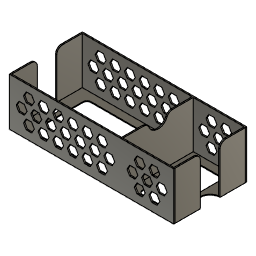
Food_Chain_Magnate_Card_Holder v2 (Autodesk Fusion 360 design; units mm, degrees)
Autodesk Fusion 360 part; units mm, degrees
sketch "Sketch1" plane through (0, 0, 0) normal (0, 0, 1) x (1, 0, 0)
  line L0 (-50, 26.6) -> (160, 26.6)
  line L1 (-50, 26.6) -> (-50, 25)
  line L2 (160, 26.6) -> (160, 25)
  line L3 (159.9999, -66.6) -> (-50, -66.6)
  line L4 (-50, -66.6) -> (-50, -65)
  line L5 (159.9999, -66.6) -> (160, -65)
  line L6 (-48.4, -64.9241) -> (-48.4, -65)
  line L7 (93.4, 25) -> (93.4, -65)
  line L8 (91.8, 25) -> (91.8, -65)
  line L9 (-48.4, 25) -> (91.8, 25)
  line L10 (93.4, 25) -> (158.4, 25)
  line L11 (158.4, -65) -> (93.4, -65)
  line L12 (91.8, -65) -> (-48.4, -65)
  line L13 (103.4, 10) -> (103.4, -50)
  line L14 (137.4, -55) -> (108.4, -55)
  line L15 (108.4, 15) -> (137.4, 15)
  line L16 (76.8, -55) -> (-27.4, -55)
  line L17 (81.8, 10) -> (81.8, -50)
  line L18 (-27.4, 15) -> (76.8, 15)
  line L19 (-32.4, 10) -> (-32.4, -50)
  line L20 (142.4, 10) -> (142.4, -50)
  arc A0 (-50, -32.5) -> (-50, -7.5) centre (-50, -20) ccw
  line L21 (-50, -65) -> (-50, -32.5)
  line L22 (-50, -7.5) -> (-50, 25)
  line L23 (-48.4, 25) -> (-48.4, -7.6028)
  line L24 (-48.4, -32.3972) -> (-48.4, -65)
  arc A1 (160, -7.5) -> (160, -32.5) centre (160, -20) ccw
  line L25 (160, 25) -> (160, -7.5)
  line L26 (160, -32.5) -> (160, -65)
  line L27 (158.4, 25) -> (158.4, -7.6028)
  line L28 (158.4, -32.3972) -> (158.4, -65)
  arc A2 (-27.4, 15) -> (-32.4, 10) centre (-27.4, 10) ccw
  arc A3 (-32.4, -50) -> (-27.4, -55) centre (-27.4, -50) ccw
  arc A4 (76.8, -55) -> (81.8, -50) centre (76.8, -50) ccw
  arc A5 (81.8, 10) -> (76.8, 15) centre (76.8, 10) ccw
  arc A6 (108.4, 15) -> (103.4, 10) centre (108.4, 10) ccw
  arc A7 (142.4, 10) -> (137.4, 15) centre (137.4, 10) ccw
  arc A8 (137.4, -55) -> (142.4, -50) centre (137.4, -50) ccw
  arc A9 (103.4, -50) -> (108.4, -55) centre (108.4, -50) ccw
  dimension "d1" = 210
  dimension "d2" = 90
  dimension "d5" = 1.6
  dimension "d6" = 1.6
  dimension "d10" = 1.6
  dimension "d11" = 1.6
  dimension "d12" = 65
  dimension "d13" = 1.6
  dimension "d16" = 16
  dimension "d17" = 16
  dimension "d18" = 25
  dimension "d19" = 25
  dimension "d24" = 5
  constraint horizontal L9
  constraint vertical L25
  constraint horizontal L11
  constraint vertical L21
  constraint perpendicular L11 L23
  constraint perpendicular L11 L27
  constraint horizontal L0
  constraint perpendicular L3 L25
  constraint coincident L6.start L23
  constraint perpendicular L6 L11
  constraint coincident L7.start L9
  constraint perpendicular L7 L11
  constraint coincident L8.end L11
  constraint perpendicular L8 L11
  constraint collinear L9 L10
  constraint collinear L11 L12
  constraint parallel L7 L13
  constraint parallel L11 L14
  constraint parallel L10 L15
  constraint parallel L12 L16
  constraint parallel L8 L17
  constraint parallel L9 L18
  constraint perpendicular L16 L19
  constraint perpendicular L14 L20
  constraint coincident A0.end L21
  constraint collinear L21 L22
  constraint coincident A0.centre L21
  constraint coincident A0 L23.end
  constraint coincident A0 L24.start
  constraint collinear L23 L24
  constraint coincident A1.end L25
  constraint collinear L25 L26
  constraint coincident A1.centre L25
  constraint coincident A1 L27.end
  constraint coincident A1 L28.start
  constraint collinear L27 L28
  constraint tangent L19 A2
  constraint tangent L18 A2
  constraint tangent L19 A3
  constraint tangent L16 A3
  constraint equal A2 A3
  constraint tangent L16 A4
  constraint tangent L17 A4
  constraint equal A2 A4
  constraint tangent L17 A5
  constraint tangent L18 A5
  constraint equal A2 A5
  constraint tangent L13 A6
  constraint tangent L15 A6
  constraint equal A2 A6
  constraint tangent L20 A7
  constraint tangent L15 A7
  constraint equal A2 A7
  constraint tangent L20 A8
  constraint tangent L14 A8
  constraint equal A2 A8
  constraint tangent L13 A9
  constraint tangent L14 A9
  constraint equal A2 A9
  measures "d1" distance of L1.end L2.end
  measures "d2" distance of L1.end L4.end
  measures "d5" distance of L21 L23
  measures "d6" distance of L25 L27
  measures "d10" distance of L0 L9
  measures "d11" distance of L3 L11
  measures "d12" distance of L7 L27
  measures "d13" distance of L7 L8
  measures "d16" distance of L19 L23
  measures "d17" distance of L20 L27
  measures "d18" diameter of A0
  measures "d19" diameter of A1
  measures "d24" radius of A2
extrude "Extrude1" add sketch "Sketch1" along normal blind 1 contours L6 L8 L9 L12 A0 L23 L24 | L7 L10 L11 A1 L27 L28 makes body 1 at (-43.0667, -49.1324, 0) makes body 2 at (153.0667, -49.1324, 0)
extrude "Extrude2" add sketch "Sketch1" along normal blind 61 contours L0 L1 L2 L3 L4 L5 L6 L7 L8 L9 L10 L11 L12 A0 L21 L22 L23 L24 A1 L25 L26 L27 L28 bodies 1 2
sketch "Sketch2" plane through (93.4, 0, 0) normal (1, 0, 0) x (0, 1, 0)
  line L0 (-65, 1) -> (25, 1)
  line L1 (25, 1) -> (25, 61)
  line L2 (25, 61) -> (-65, 61)
  line L3 (-65, 61) -> (-65, 1)
  arc A0 (-32.5, 61) -> (-7.5, 61) centre (-20, 61) ccw
  dimension "d27" = 25
  constraint midpoint L2 A0.centre
  constraint coincident L2 A0.end
  constraint coincident L2 A0.start
  measures "d27" diameter of A0
extrude "Extrude3" cut sketch "Sketch2" against normal blind 12 contours L2 A0 bodies 1
fillet "Fillet1" radius 7.5 6 edges at (-49.1983, -32.4743, 61) (-49.1983, -7.5257, 61) (159.1983, -7.5257, 61) (159.1983, -32.4743, 61) (92.6, -7.5, 61) (92.6, -32.5, 61) on bodies 1
sketch "Sketch3" plane through (0, -66.6, 0) normal (0, -1, 0) x (1, 0, 0)
  line L0 (-50, 0) -> (159.9999, 0)
  line L1 (159.9999, 0) -> (159.9999, 61)
  line L2 (159.9999, 61) -> (-50, 61)
  line L3 (-50, 61) -> (-50, 0)
  line L4 (-48.4, 61) -> (-48.4, 0)
  line L5 (158.3999, 61) -> (158.3999, 0)
  line L6 (93.3999, 61) -> (93.3999, 0)
  line L7 (91.7999, 61) -> (91.7999, 0)
  line L8 (-50, 1) -> (159.9999, 1)
  line L9 (18.2358, 37) -> (14.7717, 31)
  line L10 (14.7717, 31) -> (18.2358, 25)
  line L11 (18.2358, 25) -> (25.164, 25)
  line L12 (25.164, 25) -> (28.6281, 31)
  line L13 (28.6281, 31) -> (25.164, 37)
  line L14 (25.164, 37) -> (18.2358, 37)
  line L15 (70.7717, 31) -> (74.2358, 25)
  line L16 (74.2358, 25) -> (81.164, 25)
  line L17 (81.164, 25) -> (84.6281, 31)
  line L18 (84.6281, 31) -> (81.164, 37)
  line L19 (81.164, 37) -> (74.2358, 37)
  line L20 (74.2358, 37) -> (70.7717, 31)
  line L21 (52.1051, 31) -> (55.5692, 25)
  line L22 (55.5692, 25) -> (62.4974, 25)
  line L23 (62.4974, 25) -> (65.9615, 31)
  line L24 (65.9615, 31) -> (62.4974, 37)
  line L25 (62.4974, 37) -> (55.5692, 37)
  line L26 (55.5692, 37) -> (52.1051, 31)
  line L27 (33.4384, 31) -> (36.9025, 25)
  line L28 (36.9025, 25) -> (43.8307, 25)
  line L29 (43.8307, 25) -> (47.2948, 31)
  line L30 (47.2948, 31) -> (43.8307, 37)
  line L31 (43.8307, 37) -> (36.9025, 37)
  line L32 (36.9025, 37) -> (33.4384, 31)
  line L33 (-3.8949, 31) -> (-0.4308, 25)
  line L34 (-0.4308, 25) -> (6.4974, 25)
  line L35 (6.4974, 25) -> (9.9615, 31)
  line L36 (9.9615, 31) -> (6.4974, 37)
  line L37 (6.4974, 37) -> (-0.4308, 37)
  line L38 (-0.4308, 37) -> (-3.8949, 31)
  line L39 (-22.5616, 31) -> (-19.0975, 25)
  line L40 (-19.0975, 25) -> (-12.1693, 25)
  line L41 (-12.1693, 25) -> (-8.7052, 31)
  line L42 (-8.7052, 31) -> (-12.1693, 37)
  line L43 (-12.1693, 37) -> (-19.0975, 37)
  line L44 (-19.0975, 37) -> (-22.5616, 31)
  line L45 (-41.2283, 31) -> (-37.7642, 25)
  line L46 (-37.7642, 25) -> (-30.836, 25)
  line L47 (-30.836, 25) -> (-27.3719, 31)
  line L48 (-27.3719, 31) -> (-30.836, 37)
  line L49 (-30.836, 37) -> (-37.7642, 37)
  line L50 (-37.7642, 37) -> (-41.2283, 31)
  line L51 (122.4358, 37) -> (118.9717, 31)
  line L52 (118.9717, 31) -> (122.4358, 25)
  line L53 (122.4358, 25) -> (129.364, 25)
  line L54 (129.364, 25) -> (132.8281, 31)
  line L55 (132.8281, 31) -> (129.364, 37)
  line L56 (129.364, 37) -> (122.4358, 37)
  line L57 (14.7717, 31) -> (9.9615, 31)
  line L58 (12.3666, 31) -> (12.3666, 46)
  line L59 (8.9025, 52) -> (5.4384, 46)
  line L60 (5.4384, 46) -> (8.9025, 40)
  line L61 (8.9025, 40) -> (15.8307, 40)
  line L62 (15.8307, 40) -> (19.2948, 46)
  line L63 (19.2948, 46) -> (15.8307, 52)
  line L64 (15.8307, 52) -> (8.9025, 52)
  line L65 (12.3666, 31) -> (12.3666, 16)
  line L66 (15.8307, 10) -> (19.2948, 16)
  line L67 (19.2948, 16) -> (15.8307, 22)
  line L68 (15.8307, 22) -> (8.9025, 22)
  line L69 (8.9025, 22) -> (5.4384, 16)
  line L70 (5.4384, 16) -> (8.9025, 10)
  line L71 (8.9025, 10) -> (15.8307, 10)
  line L72 (27.5692, 22) -> (24.1051, 16)
  line L73 (24.1051, 16) -> (27.5692, 10)
  line L74 (27.5692, 10) -> (34.4974, 10)
  line L75 (34.4974, 10) -> (37.9615, 16)
  line L76 (37.9615, 16) -> (34.4974, 22)
  line L77 (34.4974, 22) -> (27.5692, 22)
  line L78 (46.2358, 22) -> (42.7717, 16)
  line L79 (42.7717, 16) -> (46.2358, 10)
  line L80 (46.2358, 10) -> (53.164, 10)
  line L81 (53.164, 10) -> (56.6281, 16)
  line L82 (56.6281, 16) -> (53.164, 22)
  line L83 (53.164, 22) -> (46.2358, 22)
  line L84 (64.9025, 22) -> (61.4384, 16)
  line L85 (61.4384, 16) -> (64.9025, 10)
  line L86 (64.9025, 10) -> (71.8307, 10)
  line L87 (71.8307, 10) -> (75.2948, 16)
  line L88 (75.2948, 16) -> (71.8307, 22)
  line L89 (71.8307, 22) -> (64.9025, 22)
  line L90 (-13.2283, 16) -> (-9.7642, 10)
  line L91 (-9.7642, 22) -> (-13.2283, 16)
  line L92 (-2.836, 22) -> (-9.7642, 22)
  line L93 (0.6281, 16) -> (-2.836, 22)
  line L94 (-2.836, 10) -> (0.6281, 16)
  line L95 (-9.7642, 10) -> (-2.836, 10)
  line L96 (-31.8949, 16) -> (-28.4308, 10)
  line L97 (-28.4308, 22) -> (-31.8949, 16)
  line L98 (-21.5026, 22) -> (-28.4308, 22)
  line L99 (-18.0385, 16) -> (-21.5026, 22)
  line L100 (-21.5026, 10) -> (-18.0385, 16)
  line L101 (-28.4308, 10) -> (-21.5026, 10)
  line L102 (-2.836, 40) -> (0.6281, 46)
  line L103 (-9.7642, 52) -> (-13.2283, 46)
  line L104 (-18.0385, 46) -> (-21.5026, 52)
  line L105 (-21.5026, 40) -> (-18.0385, 46)
  line L106 (34.4974, 40) -> (37.9615, 46)
  line L107 (37.9615, 46) -> (34.4974, 52)
  line L108 (61.4384, 46) -> (64.9025, 40)
  line L109 (15.8307, 40) -> (19.2948, 46)
  line L110 (71.8307, 52) -> (64.9025, 52)
  line L111 (8.9025, 40) -> (15.8307, 40)
  line L112 (27.5692, 52) -> (24.1051, 46)
  line L113 (56.6281, 46) -> (53.164, 52)
  line L114 (64.9025, 52) -> (61.4384, 46)
  line L115 (46.2358, 52) -> (42.7717, 46)
  line L116 (19.2948, 46) -> (15.8307, 52)
  line L117 (-2.836, 52) -> (-9.7642, 52)
  line L118 (46.2358, 40) -> (53.164, 40)
  line L119 (-21.5026, 52) -> (-28.4308, 52)
  line L120 (75.2948, 46) -> (71.8307, 52)
  line L121 (-28.4308, 40) -> (-21.5026, 40)
  line L122 (-13.2283, 46) -> (-9.7642, 40)
  line L123 (71.8307, 40) -> (75.2948, 46)
  line L124 (53.164, 52) -> (46.2358, 52)
  line L125 (64.9025, 40) -> (71.8307, 40)
  line L126 (-9.7642, 40) -> (-2.836, 40)
  line L127 (8.9025, 52) -> (5.4384, 46)
  line L128 (24.1051, 46) -> (27.5692, 40)
  line L129 (34.4974, 52) -> (27.5692, 52)
  line L130 (5.4384, 46) -> (8.9025, 40)
  line L131 (53.164, 40) -> (56.6281, 46)
  line L132 (0.6281, 46) -> (-2.836, 52)
  line L133 (27.5692, 40) -> (34.4974, 40)
  line L134 (42.7717, 46) -> (46.2358, 40)
  line L135 (15.8307, 52) -> (8.9025, 52)
  line L136 (-31.8949, 46) -> (-28.4308, 40)
  line L137 (-28.4308, 52) -> (-31.8949, 46)
  line L138 (118.9717, 31) -> (114.1707, 31)
  line L139 (114.1707, 31) -> (107.2427, 31)
  line L140 (103.7786, 37) -> (100.3144, 31)
  line L141 (100.3144, 31) -> (103.7786, 25)
  line L142 (103.7786, 25) -> (110.7068, 25)
  line L143 (110.7068, 25) -> (114.1709, 31)
  line L144 (114.1709, 31) -> (110.7068, 37)
  line L145 (110.7068, 37) -> (103.7786, 37)
  line L146 (132.8281, 31) -> (137.6291, 31)
  line L147 (137.6291, 31) -> (144.5571, 31)
  line L148 (141.093, 37) -> (137.6289, 31)
  line L149 (137.6289, 31) -> (141.093, 25)
  line L150 (141.093, 25) -> (148.0212, 25)
  line L151 (148.0212, 25) -> (151.4853, 31)
  line L152 (151.4853, 31) -> (148.0212, 37)
  line L153 (148.0212, 37) -> (141.093, 37)
  line L154 (116.5712, 31) -> (116.5712, 46)
  line L155 (116.5712, 31) -> (116.5712, 16)
  line L156 (135.2286, 31) -> (135.2286, 46)
  line L157 (135.2286, 31) -> (135.2286, 16)
  line L158 (131.7645, 52) -> (128.3004, 46)
  line L159 (128.3004, 46) -> (131.7645, 40)
  line L160 (131.7645, 40) -> (138.6927, 40)
  line L161 (138.6927, 40) -> (142.1568, 46)
  line L162 (142.1568, 46) -> (138.6927, 52)
  line L163 (138.6927, 52) -> (131.7645, 52)
  line L164 (113.1071, 52) -> (109.6429, 46)
  line L165 (109.6429, 46) -> (113.1071, 40)
  line L166 (113.1071, 40) -> (120.0353, 40)
  line L167 (120.0353, 40) -> (123.4994, 46)
  line L168 (123.4994, 46) -> (120.0353, 52)
  line L169 (120.0353, 52) -> (113.1071, 52)
  line L170 (120.0353, 10) -> (123.4994, 16)
  line L171 (123.4994, 16) -> (120.0353, 22)
  line L172 (120.0353, 22) -> (113.1071, 22)
  line L173 (113.1071, 22) -> (109.6429, 16)
  line L174 (109.6429, 16) -> (113.1071, 10)
  line L175 (113.1071, 10) -> (120.0353, 10)
  line L176 (138.6927, 10) -> (142.1568, 16)
  line L177 (142.1568, 16) -> (138.6927, 22)
  line L178 (138.6927, 22) -> (131.7645, 22)
  line L179 (131.7645, 22) -> (128.3004, 16)
  line L180 (128.3004, 16) -> (131.7645, 10)
  line L181 (131.7645, 10) -> (138.6927, 10)
  point P0 (12.3666, 46)
  point P1 (12.3666, 16)
  point P2 (12.3666, 46)
  point P3 (12.3666, 46)
  point P4 (114.1707, 46)
  point P5 (114.1707, 16)
  point P6 (107.2427, 31)
  point P7 (144.5571, 31)
  point P8 (135.2286, 46)
  point P9 (116.5712, 46)
  point P10 (116.5712, 16)
  point P11 (135.2286, 16)
  dimension "d30" = 1.6
  dimension "d31" = 1.6
  dimension "d32" = 65
  dimension "d33" = 1.6
  dimension "d34" = 1
  dimension "d38" = -56
  dimension "d39" = 0
  dimension "d47" = 6
  dimension "d48" = 15
  dimension "d49" = 6
  dimension "d56" = 56
  dimension "d57" = 0
  dimension "d60" = -56
  dimension "d61" = 0
  dimension "d64" = 0
  dimension "d65" = 30
  dimension "d66" = 4.801
  dimension "d67" = 15
  dimension "d68" = 15
  dimension "d71" = 6.928
  dimension "d72" = 6
  dimension "d73" = 4.801
  dimension "d76" = 6.928
  dimension "d77" = 6
  dimension "d78" = 15
  dimension "d79" = 15
  dimension "d80" = 15
  dimension "d81" = 15
  dimension "d82" = 6
  dimension "d83" = 6
  dimension "d84" = 6
  dimension "d85" = 6
  constraint coincident L2 L4.start
  constraint coincident L0 L4.end
  constraint perpendicular L0 L4
  constraint coincident L2 L5.start
  constraint coincident L0 L5.end
  constraint perpendicular L0 L5
  constraint coincident L2 L6.start
  constraint coincident L0 L6.end
  constraint perpendicular L0 L6
  constraint coincident L2 L7.start
  constraint coincident L0 L7.end
  constraint perpendicular L0 L7
  constraint coincident L3 L8.start
  constraint coincident L1 L8.end
  constraint perpendicular L1 L8
  constraint horizontal L57
  constraint midpoint L57 L58.start
  constraint perpendicular L57 L58
  constraint coincident P3 P2
  constraint perpendicular L57 L65
  constraint coincident P1 L65.end
  constraint horizontal L138
  constraint coincident P6 L139.end
  constraint horizontal L146
  constraint coincident P7 L147.end
  constraint midpoint L138 L154.start
  constraint perpendicular L138 L154
  constraint perpendicular L138 L155
  constraint midpoint L146 L156.start
  constraint perpendicular L146 L156
  constraint perpendicular L146 L157
  constraint coincident P8 L156.end
  constraint coincident P9 L154.end
  constraint coincident P10 L155.end
  constraint coincident P11 L157.end
  measures "d30" distance of L3 L4
  measures "d31" distance of L1 L5
  measures "d32" distance of L5 L6
  measures "d33" distance of L6 L7
  measures "d34" distance of L0 L8
  measures "d47" distance of P3 L64
  measures "d48" distance of L58.start P1
  measures "d49" distance of P1 L71
  measures "d66" distance of L51.end L138.end
  measures "d67" distance of L138.end P5
  measures "d68" distance of L138.end P4
  measures "d71" distance of L138.end P6
  measures "d72" distance of P6 L145
  measures "d73" distance of L54.end L146.end
  measures "d76" distance of L146.end P7
  measures "d77" distance of P7 L153
  measures "d78" distance of L154.start P9
  measures "d79" distance of L154.start P10
  measures "d80" distance of L156.start P8
  measures "d81" distance of L156.start P11
  measures "d82" distance of P8 L163
  measures "d83" distance of P9 L169
  measures "d84" distance of P10 L175
  measures "d85" distance of P11 L181
extrude "Extrude4" cut sketch "Sketch3" against normal blind 145 contours L9 L10 L11 L12 L13 L14 | L15 L16 L17 L18 L19 L20 | L21 L22 L23 L24 L25 L26 | L27 L28 L29 L30 L31 L32 | L33 L34 L35 L36 L37 L38 | L39 L40 L41 L42 L43 L44 | L45 L46 L47 L48 L49 L50 | L51 L52 L53 L54 L55 L56 | L59 L60 L61 L62 L63 L64 L109 L111 L116 L127 L130 L135 | L66 L67 L68 L69 L70 L71 | L72 L73 L74 L75 L76 L77 | L78 L79 L80 L81 L82 L83 | L84 L85 L86 L87 L88 L89 | L90 L91 L92 L93 L94 L95 | L96 L97 L98 L99 L100 L101 | L102 L103 L117 L122 L126 L132 | L104 L105 L119 L121 L136 L137 | L106 L107 L112 L128 L129 L133 | L108 L110 L114 L120 L123 L125 | L113 L115 L118 L124 L131 L134 | L140 L141 L142 L143 L144 L145 | L148 L149 L150 L151 L152 L153 | L158 L159 L160 L161 L162 L163 | L164 L165 L166 L167 L168 L169 | L170 L171 L172 L173 L174 L175 | L176 L177 L178 L179 L180 L181 bodies 1
